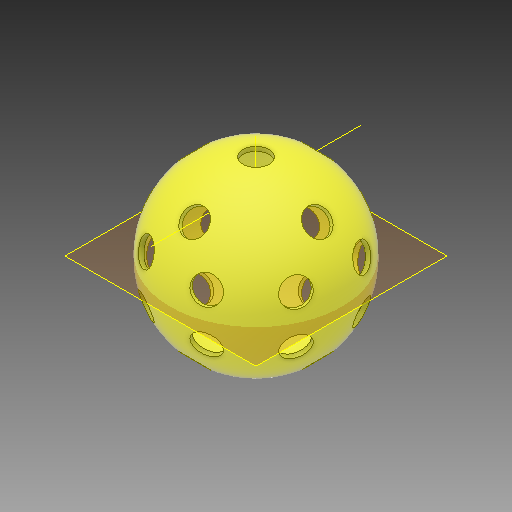
# Autodesk Inventor part: Ball
Saved by Autodesk Inventor 2017 SP1 (Build 210196100, 196)
## iProperties
Category: Ball
Company: Autodesk Inc.
Created: 2017-01-04
Part Number: Ball
Material: Polyethylene, High Density
Document SubType Name: Modeling
Designer: Autodesk Inc.
Density: 0.952 g/cm^3
Appearance: Smooth - Yellow
Catalog Web Link: http://www.gophersport.com/sports/baseball/resisdent-balls?ca=2001#
Vendor: Gopher
Mass: 123.094 g
Surface Area: 864.909 cm^2
Volume: 129.3 cm^3
Author: Autodesk Inc.
Autodesk Inventor part; units mm, degrees
sketch "Sketch1" plane through (0, 0, 0) normal (0, 1, 0) x (-1, 0, 0)
  arc A0 (-63.5, 0) -> (63.5, 0) centre (0, 0) ccw
  line L0 (63.5, 0) -> (-63.5, 0)
  arc A1 (-60.325, 0) -> (60.325, 0) centre (0, 0) ccw
  dimension "d0" = 127
  dimension "d5" = 3.175
  constraints: 4 point on circle, 2 centre point, 2 end point, 2 point on line, 1 coincident, 1 horizontal
  measures "d0" diameter of A0
  measures "d5" radial gap between concentric circles of A0 A1
revolve "Revolution2" add sketch "Sketch1" angle 360 about axis through (-63.5, 0, 0) along (1, 0, 0) contours L0 A1 A0
ref_plane "Work Plane2" through (0, 0, 63.5) normal (0, 0, 1) x (1, 0, 0)
sketch "Sketch3" plane through (0, 0, 63.5) normal (0, 0, 1) x (1, 0, 0)
  circle A0 centre (0, 0) radius 9.525
  dimension "d7" = 19.05
  constraints: 1 centre point, 1 coincident
  measures "d7" diameter of A0
extrude "Extrusion2" cut sketch "Sketch3" against normal through all
ref_plane "Work Plane3" through (0, 0, 44.45) normal (0, 0, 1) x (1, 0, 0)
sketch "Sketch4" plane through (0, 0, 44.45) normal (0, 0, 1) x (1, 0, 0)
  line L0 (88.9, 0) -> (-88.9, 0) projected
  circle A0 centre (0, 0) radius 40.7836 projected
  circle A1 centre (0, 0) radius 45.3481 projected
  point P0 (45.3481, 0)
  point P1 (45.3481, 0)
  constraints: 2 point on circle
ref_plane "Work Plane4" through (45.3481, 0, 44.45) normal (0.7141428, 0, 0.7) x (0, 1, 0)
sketch "Sketch5" plane through (45.3481, 0, 44.45) normal (0.7141428, 0, 0.7) x (0, 1, 0)
  circle A0 centre (0, 0) radius 9.525
  point P0 (0, 0)
  dimension "d11" = 19.05
  constraints: 1 centre point, 1 coincident
  measures "d11" diameter of A0
extrude "Extrusion3" cut sketch "Sketch5" against normal up to next
pattern_circular "Circular Pattern1" count 4 over 360 about axis through (0, 0, -10) along (0, 0, 1) of "Extrusion3"
ref_plane "Work Plane5" through (0, 0, 17.4625) normal (0, 0, 1) x (1, 0, 0)
ref_plane "Work Plane6" through (0, 0, 0) normal (-0.3420201, 0.9396926, 0) x (0, 0, 1)
sketch "Sketch6" plane through (0, 0, 17.4625) normal (0, 0, 1) x (1, 0, 0)
  circle A0 centre (0, 0) radius 57.7422 projected
  circle A1 centre (0, 0) radius 61.0517 projected
  line L0 (-107.0726, -38.9712) -> (107.0726, 38.9712) projected
  point P0 (-57.3698, -20.8809)
  constraints: 1 point on line, 2 other
ref_plane "Work Plane7" through (-57.3698, -20.8809, 17.4625) normal (-0.903462, -0.3288333, 0.275) x (0.3420201, -0.9396926, 0)
sketch "Sketch7" plane through (-57.3698, -20.8809, 17.4625) normal (-0.903462, -0.3288333, 0.275) x (0.3420201, -0.9396926, 0)
  circle A0 centre (0, 0) radius 9.525
  point P0 (0, 0)
  dimension "d19" = 19.05
  constraints: 1 centre point, 1 coincident
  measures "d19" diameter of A0
extrude "Extrusion4" cut sketch "Sketch7" against normal up to next
pattern_circular "Circular Pattern2" count 8 over 360 about axis through (0, 0, -10) along (0, 0, 1) of "Extrusion4"
mirror "Mirror1" about plane through (0, 0, 0) normal (0, 0, 1) of "Extrusion3", "Circular Pattern1"
mirror "Mirror2" about plane through (0, 0, 0) normal (0, 0, 1) of "Extrusion4", "Circular Pattern2"
body "Solid1"
body "Solid2"
